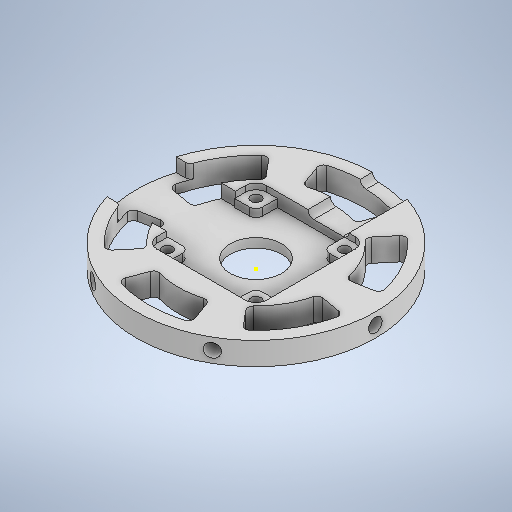
# Autodesk Inventor part: oDrive_micro_housing
Saved by Autodesk Inventor 2025.2 (Build 292293000, 293)
## iProperties
Created: 2025-04-12
Part Number: oDrive_micro_housing
Material: Generic
Document SubType Name: Modeling
Designer: Bruno
Density: 1 g/cm^3
Appearance: Default
Author: Bruno
Autodesk Inventor part; units mm, degrees
ref_plane "XZ Plane" through (0, 0, 0) normal (0, 1, 0) x (-1, 0, 0)
ref_plane "XY Plane" through (0, 0, 0) normal (0, 0, 1) x (1, 0, 0)
sketch "Sketch1" plane through (0, 0, 0) normal (0, 1, 0) x (-1, 0, 0)
  circle A0 centre (0, 0) radius 35.25 construction
  circle A1 centre (0, 0) radius 35.15
  dimension "d0" = 70.5
  dimension "d1" = 0.1
  constraints: 2 centre point, 2 coincident
  measures "d0" diameter of A0
  measures "d1" radial gap between concentric circles of A1 A0
extrude "Extrusion1" add sketch "Sketch1" along normal blind 6.7
sketch "Sketch2" plane through (0, 6.7, 0) normal (0, 1, 0) x (1, 0, 0)
  circle A0 centre (0, 0) radius 35.15 projected
  circle A1 centre (0, 0) radius 7.575
  dimension "d4" = 15.15
  constraints: 1 centre point, 1 coincident
  measures "d4" diameter of A1
extrude "Extrusion2" cut sketch "Sketch2" against normal through all contours A1
sketch "Sketch3" plane through (0, 6.7, 0) normal (0, 1, 0) x (1, 0, 0)
  line L0 (-13, -16.15) -> (13, -16.15)
  line L1 (16.15, -13) -> (16.15, 13)
  line L2 (13, 16.15) -> (-13, 16.15)
  circle A0 centre (0, 0) radius 7.575 projected
  line L3 (-16.15, -16.15) -> (16.15, 16.15) construction
  line L4 (16.15, -16.15) -> (-16.15, 16.15) construction
  line L5 (-13, -13) -> (13, -13) construction
  line L6 (13, -13) -> (13, 13) construction
  line L7 (13, 13) -> (-13, 13) construction
  line L8 (-13, 13) -> (-13, -13) construction
  line L9 (-13, -13) -> (13, 13) construction
  line L10 (13, -13) -> (-13, 13) construction
  arc A1 (-16.15, -13) -> (-13, -16.15) centre (-13, -13) ccw
  arc A2 (13, -16.15) -> (16.15, -13) centre (13, -13) ccw
  arc A3 (16.15, 13) -> (13, 16.15) centre (13, 13) ccw
  arc A4 (-13, 16.15) -> (-16.15, 13) centre (-13, 13) ccw
  line L11 (-16.15, -10.15) -> (-33.6526, -10.15)
  circle A5 centre (0, 0) radius 35.15 projected
  line L12 (-35.15, 0) -> (-16.15, 0) construction
  circle A6 centre (0, 0) radius 35.15 projected
  line L13 (-16.15, 10.15) -> (-33.6526, 10.15)
  line L14 (-16.15, 13) -> (-16.15, 10.15)
  line L15 (-16.15, -10.15) -> (-16.15, -13)
  dimension "d7" = 32.3
  dimension "d8" = 32.3
  dimension "d9" = 26
  dimension "d10" = 26
  dimension "d11" = 3.15
  dimension "d14" = 20.3
  constraints: 32 end point, 9 point on circle, 7 tangent, 5 horizontal, 5 parallel, 4 centre point, 4 coincident, 4 midpoint, 2 perpendicular, 2 symmetric about line, 2 other
  measures "d7" distance of L4.end L3.end
  measures "d8" distance of L3.end L4.start
  measures "d9" distance of L7.end L6.end
  measures "d10" distance of L6.end L5.end
  measures "d11" radius of A1
  measures "d14" diameter of L11 L12
extrude "Extrusion3" cut sketch "Sketch3" against normal blind 4 contours A1 L15 L11 A5 L13 L14 A4 L2 A3 L1 A2 L0 picked at (-22.4275, 1.1423)
sketch "Sketch4" plane through (0, 2.7, 0) normal (0, 1, 0) x (1, 0, 0)
  line L0 (-33.6526, 10.15) -> (-16.15, 10.15) projected
  arc A0 (-33.6526, 10.15) -> (-33.6526, -10.15) centre (0, 0) ccw projected
  line L1 (-16.15, -10.15) -> (-33.6526, -10.15) projected
  line L2 (-16.15, -13) -> (-16.15, -10.15) projected
  arc A1 (-16.15, -13) -> (-13, -16.15) centre (-13, -13) ccw projected
  line L3 (13, -16.15) -> (-13, -16.15) projected
  arc A2 (13, -16.15) -> (16.15, -13) centre (13, -13) ccw projected
  line L4 (16.15, 13) -> (16.15, -13) projected
  arc A3 (16.15, 13) -> (13, 16.15) centre (13, 13) ccw projected
  line L5 (-13, 16.15) -> (13, 16.15) projected
  arc A4 (-13, 16.15) -> (-16.15, 13) centre (-13, 13) ccw projected
  line L6 (-16.15, 10.15) -> (-16.15, 13) projected
  circle A5 centre (0, 0) radius 7.575 projected
  circle A6 centre (-13, -13) radius 1.5
  circle A7 centre (-13, 13) radius 1.5
  circle A8 centre (13, -13) radius 1.5
  circle A9 centre (13, 13) radius 1.5
  line L7 (-9.85, -16.15) -> (-9.85, -9.85)
  line L8 (-9.85, -9.85) -> (-16.15, -9.85)
  line L9 (-16.15, -9.85) -> (-16.15, -10.15)
  line L10 (-13, -13) -> (-13, -16.15) construction
  line L11 (-13, -13) -> (-13, -9.85) construction
  line L12 (0, 0) -> (3.189, 0) construction
  line L13 (0, 0) -> (0, 2.3999) construction
  line L14 (-9.85, 16.15) -> (-9.85, 9.85)
  line L15 (-9.85, 9.85) -> (-16.15, 9.85)
  line L16 (-16.15, 9.85) -> (-16.15, 10.15)
  line L17 (9.85, -16.15) -> (9.85, -9.85)
  line L18 (9.85, -9.85) -> (16.15, -9.85)
  line L19 (9.85, 9.85) -> (16.15, 9.85)
  line L20 (9.85, 16.15) -> (9.85, 9.85)
  dimension "d17" = 3
  dimension "d18" = 3
  dimension "d19" = 3
  dimension "d20" = 3
  constraints: 28 end point, 9 symmetric about line, 5 vertical, 4 centre point, 4 coincident, 2 equal length, 2 perpendicular, 1 horizontal, 1 midpoint, 1 point on line
  measures "d17" diameter of A6
  measures "d18" diameter of A7
  measures "d19" diameter of A8
  measures "d20" diameter of A9
extrude "Extrusion4" add sketch "Sketch4" along normal blind 2.3 contours L6 A4 L5 L14 L15 L16 | L9 L8 L7 L3 A1 L2 | L5 A3 L4 L19 L20 | L17 L18 L4 A2 L3
fillet "Fillet1" radius 2 4 edges at (-9.85, 3.85, 9.85) (-9.85, 3.85, -9.85) (9.85, 3.85, -9.85) (9.85, 3.85, 9.85)
sketch "Sketch5" plane through (0, 6.7, 0) normal (0, 1, 0) x (1, 0, 0)
  line L0 (9.85, 16.15) -> (13, 16.15) projected
  line L1 (11.15, 16.15) -> (11.15, 33.3347)
  circle A0 centre (0, 0) radius 35.15 projected
  line L2 (-0.85, 16.15) -> (-0.85, 35.1397)
  line L3 (-9.85, 16.15) -> (9.85, 16.15) projected
  line L4 (-13, 16.15) -> (13, 16.15) projected
  arc A1 (-33.6526, -10.15) -> (-33.6526, 10.15) centre (0, 0) ccw projected
  line L5 (16.15, 13) -> (16.15, -13) projected
  dimension "d24" = 12
  dimension "d25" = 5
  constraints: 4 end point, 2 point on circle, 2 point on line, 1 perpendicular, 1 vertical
  measures "d24" distance between parallel lines of L2 L1
  measures "d25" distance between parallel lines of L5 L1
extrude "Extrusion5" cut sketch "Sketch5" against normal up to surface (1.7 mm away) contours L3 L2 A0 L1 L0 picked at (5.4096, 22.2329)
fillet "Fillet2" radius 1.7 2 edges at (11.15, 5, -24.7423) (-0.85, 5, -25.6449)
sketch "Sketch6" plane through (0, 0, 0) normal (0, 1, 0) x (-1, 0, 0)
  point P0 (0, 0)
ref_plane "Work Plane2" through (-17.575, 0, -30.4408) normal (0.5, 0, 0.8660254) x (0, 1, 0)
ref_plane "Work Plane1" through (0, 0, 0) normal (0.5, 0, 0.8660254) x (0, 1, 0)
sketch "Sketch7" plane through (-17.575, 0, -30.4408) normal (0.5, 0, 0.8660254) x (0, 1, 0)
  line L0 (6.7, -16.8337) -> (6.7, 24.069) projected
  circle A0 centre (3.35, 0) radius 2
  line L1 (-1.3403, 0) -> (8.0418, 0) construction
  line L2 (6.7, 0) -> (3.35, 0)
  line L3 (3.35, 0) -> (0, 0)
  dimension "d30" = 4
  constraints: 4 end point, 2 collinear, 2 point on line, 1 centre point, 1 horizontal
  measures "d30" diameter of A0
extrude "Extrusion6" cut sketch "Sketch7" along normal blind 7
pattern_circular "Circular Pattern1" count 5 over 240 about axis through (0, 0, 0) along (0, -1, 0) of "Extrusion6"
sketch "Sketch8" plane through (0, 6.7, 0) normal (0, 1, 0) x (1, 0, 0)
  arc A0 (-33.6526, -10.15) -> (11.15, 33.3347) centre (0, 0) ccw projected
  circle A1 centre (0, 0) radius 31.55
  circle A2 centre (0, 0) radius 22.7348
  arc A3 (-13, 16.15) -> (-16.15, 13) centre (-13, 13) ccw projected
  line L0 (0, 0) -> (-31.0707, 5.4786)
  line L1 (0, 0) -> (-31.0707, -5.4786)
  line L2 (0, 0) -> (-5.4003, 0) construction
  line L3 (0, 0) -> (-10.7907, -29.6473)
  line L4 (0, 0) -> (-20.2799, -24.1687)
  line L5 (0, 0) -> (20.2799, -24.1687)
  line L6 (0, 0) -> (10.7907, -29.6473)
  line L7 (0, 0) -> (31.0707, 5.4786)
  line L8 (0, 0) -> (31.0707, -5.4786)
  line L9 (0, 0) -> (10.7907, 29.6473)
  line L10 (0, 0) -> (20.2799, 24.1687)
  line L11 (0, 0) -> (-20.2799, 24.1687)
  line L12 (0, 0) -> (-10.7907, 29.6473)
  point P0 (-14.6136, 17.4158)
  point P1 (-20.2799, 24.1687)
  point P2 (-22.3894, 3.9479)
  point P3 (-10.7907, 29.6473)
  point P4 (-7.7758, 21.3637)
  point P5 (7.7758, 21.3637)
  point P6 (10.7907, 29.6473)
  point P7 (20.2799, 24.1687)
  point P8 (14.6136, 17.4158)
  point P9 (22.3894, 3.9479)
  point P10 (31.0707, 5.4786)
  point P11 (31.0707, -5.4786)
  point P12 (22.3894, -3.9479)
  point P13 (14.6136, -17.4158)
  point P14 (20.2799, -24.1687)
  point P15 (10.7907, -29.6473)
  point P16 (7.7758, -21.3637)
  point P17 (-7.7758, -21.3637)
  point P18 (-10.7907, -29.6473)
  point P19 (-20.2799, -24.1687)
  point P20 (-14.6136, -17.4158)
  point P21 (-22.3894, -3.9479)
  dimension "d37" = 1.2
  dimension "d38" = 3.6
  dimension "d39" = 20
  dimension "d40" = 10
  dimension "d43" = 360
  constraints: 26 end point, 2 centre point, 2 coincident, 2 point on circle, 1 horizontal, 31 other
  measures "d38" radial gap between concentric circles of A0 A1
  measures "d39" angle of L0 L1
  measures "d40" angle of L2 L1
extrude "Extrusion7" cut sketch "Sketch8" against normal through all contours L7 A2 L10 A1 | A1 L5 A2 L8 | L9 A2 L12 A1 | A1 L3 A2 L6 | L0 A1 L11 A2 | A2 L4 A1 L1
fillet "Fillet3" radius 1.5 24 edges at (-31.0707, 1.35, 5.4786) (-20.2799, 3.35, 24.1687) (-22.3894, 1.35, 3.9479) (-14.6136, 3.35, 17.4158) (-10.7907, 3.35, 29.6473) (-7.7758, 3.35, 21.3637) (10.7907, 3.35, 29.6473) (7.7758, 3.35, 21.3637) (14.6136, 3.35, 17.4158) (20.2799, 3.35, 24.1687) (22.3894, 3.35, 3.9479) (31.0707, 3.35, 5.4786) (22.3894, 3.35, -3.9479) (14.6136, 3.35, -17.4158) (31.0707, 3.35, -5.4786) (20.2799, 3.35, -24.1687) (10.7907, 2.8274, -29.6473) (7.7758, 2.5, -21.3637) (-7.7758, 3.35, -21.3637) (-10.7907, 3.35, -29.6473) (-14.6136, 3.35, -17.4158) (-20.2799, 3.35, -24.1687) (-31.0707, 1.35, -5.4786) (-22.3894, 1.35, -3.9479)
fillet "Fillet4" radius 1.5 2 edges at (-29.8727, 4.7, 10.15) (-29.8727, 4.7, -10.15)
equation "\"d40\" = 0.5 * d39"
body "Solid1"
